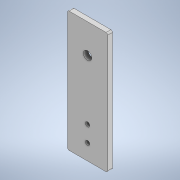
# Autodesk Inventor part: Columna
Saved by Autodesk Inventor 2022 (Build 260153000, 153)
## iProperties
Created: 2022-02-04
Part Number: Columna
Material: Generic
Document SubType Name: Modeling
Designer: Home
Density: 1 g/cm^3
Appearance: Default
Author: Home
Autodesk Inventor part; units mm, degrees
ref_plane "YZ Plane" through (0, 0, 0) normal (1, 0, 0) x (0, 1, 0)
ref_plane "XZ Plane" through (0, 0, 0) normal (0, 1, 0) x (-1, 0, 0)
ref_plane "XY Plane" through (0, 0, 0) normal (0, 0, 1) x (1, 0, 0)
sketch "Sketch2" plane through (0, 0, 0) normal (0, 0, 1) x (1, 0, 0)
  line L0 (-25, 75) -> (25, 75)
  line L1 (25, 75) -> (25, -75)
  line L2 (25, -75) -> (-25, -75)
  line L3 (-25, -75) -> (-25, 75)
  line L4 (-25, 75) -> (25, -75) construction
  line L5 (25, 75) -> (-25, -75) construction
  point P0 (0, 0)
  dimension "d0" = 50
  dimension "d1" = 150
  constraints: 12 end point, 2 midpoint, 2 parallel, 1 horizontal, 1 perpendicular
  measures "d0" distance of L1.end L2.end
  measures "d1" distance of L2.end L0.start
extrude "Extrusion1" add sketch "Sketch2" along normal blind 6
fillet "Fillet1" radius 2 4 edges at (25, 75, 3) (-25, 75, 3) (25, -75, 3) (-25, -75, 3)
sketch "Sketch3" plane through (0, 0, 6) normal (0, 0, 1) x (1, 0, 0)
  line L0 (23, 75) -> (-23, 75) projected
  point P0 (0, 0)
  point P1 (0, 38.6)
  point P2 (0, 75)
  dimension "d5" = 36.4
  constraints: 1 midpoint, 1 vertical alignment
  measures "d5" distance from line of point (0, 38.6) L0
hole "Hole1" at (0, 38.6, 6) direction (0, 0, -1) diameter 10.5 end through all
sketch "Sketch4" plane through (0, 0, 6) normal (0, 0, 1) x (1, 0, 0)
  line L0 (-23, -75) -> (23, -75) projected
  point P0 (0, 0)
  point P1 (0, -55.449)
  point P2 (0, -35.449)
  dimension "d13" = 20
  dimension "d14" = 39.551
  constraints: 2 vertical alignment
  measures "d13" distance of point (0, -35.449) point (0, -55.449)
  measures "d14" distance from line of L0 point (0, -35.449)
hole "Hole2" at (0, -55.449, 6) at (0, -35.449, 6) direction (0, 0, -1) diameter 5.4 end through all
body "Solid1"
